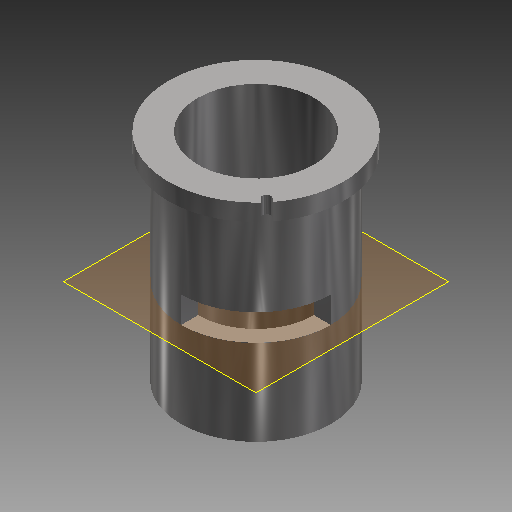
# Autodesk Inventor part: Piston Shaft
Saved by Autodesk Inventor 2017 (Build 210142000, 142)
## iProperties
Created: 2012-08-14
Part Number: Piston Shaft
Material: Stainless Steel
Document SubType Name: Modeling
Designer: John
Density: 1 g/cm^3
Appearance: Semi-Polished
Author: John
Autodesk Inventor part; units mm, degrees
ref_plane "YZ Plane" through (0, 0, 0) normal (1, 0, 0) x (0, 1, 0)
ref_plane "XZ Plane" through (0, 0, 0) normal (0, 1, 0) x (-1, 0, 0)
ref_plane "XY Plane" through (0, 0, 0) normal (0, 0, 1) x (1, 0, 0)
sketch "Sketch1" plane through (0, 0, 0) normal (0, 1, 0) x (-1, 0, 0)
  circle A0 centre (0, 0) radius 10.541
  dimension "d2" = 21.082
  constraints: 1 centre point, 1 coincident
  measures "d2" diameter of A0
extrude "Extrusion1" add sketch "Sketch1" along normal blind 2.032
sketch "Sketch2" plane through (0, 0, 0) normal (0, -1, 0) x (1, 0, 0)
  circle A0 centre (0, 0) radius 10.541 projected
  circle A1 centre (0, 0) radius 9.017
  dimension "d4" = 18.034
  constraints: 1 centre point, 1 coincident
  measures "d4" diameter of A1
extrude "Extrusion2" add sketch "Sketch2" along normal blind 24.003 contours A1
hole "Hole1" at (0, 2.032, 0) direction (0, -1, 0) diameter 13.97 end through all
ref_plane "Work Plane1" through (0, -13.6652, 0) normal (0, 1, 0) x (1, 0, 0)
sketch "Sketch3" plane through (0, -13.6652, 0) normal (0, 1, 0) x (1, 0, 0)
  line L0 (0, 0) -> (9.017, 0)
  line L1 (9.017, 0) -> (9.017, -9.017)
  line L2 (9.017, -9.017) -> (0, -9.017)
  line L3 (0, -9.017) -> (0, 0)
  dimension "d17" = 9.017
  dimension "d18" = 9.017
  constraints: 8 end point, 2 parallel, 1 horizontal, 1 perpendicular
  measures "d17" distance of L1.end L2.end
  measures "d18" distance of L0.end L1.end
extrude "Extrusion3" cut sketch "Sketch3" along normal blind 3.175
sketch "Sketch4" plane through (0, 2.032, 0) normal (0, 1, 0) x (1, 0, 0)
  circle A0 centre (0, 0) radius 10.541 projected
  circle A1 centre (7.62, -6.35) radius 0.508
  line L0 (7.62, -6.35) -> (0, 0) construction
  line L1 (7.9452, -5.9597) -> (8.4136, -6.3501)
  line L2 (7.2948, -6.7403) -> (7.7632, -7.1306)
  dimension "d21" = 1.016
  dimension "d22" = 6.35
  dimension "d23" = 7.62
  constraints: 6 end point, 4 point on circle, 2 parallel, 2 tangent, 1 centre point
  measures "d21" diameter of A1
  measures "d22" vertical distance of L0.end L0.start
  measures "d23" horizontal distance of L0.end L0.start
extrude "Extrusion4" cut sketch "Sketch4" against normal up to surface (2.032 mm away) contours L2 A1 L1 A0 | A1 picked at (8.2446, -6.4771)
body "Solid1"
